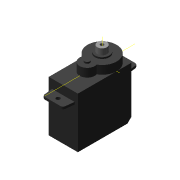
# Autodesk Inventor part: empty
Saved by Autodesk Inventor 2014 (Build 180170000, 170)
## iProperties
Created: 2015-04-13
Part Number: empty
Material: Generic
Document SubType Name: Modeling
Designer: Martin
Density: 1 g/cm^3
Appearance: Default
Author: Martin
Autodesk Inventor part; units mm, degrees
ref_plane "YZ Plane" through (0, 0, 0) normal (1, 0, 0) x (0, 1, 0)
ref_plane "XZ Plane" through (0, 0, 0) normal (0, 1, 0) x (-1, 0, 0)
sketch "Sketch1" plane through (0, 0, 0) normal (0, 0, 1) x (1, 0, 0)
  line L0 (-8.12, 0) -> (8.12, 0) projected
  line L1 (0, -19.7) -> (0, 10.05) projected
  circle A0 centre (0, 0) radius 5.8
  line L2 (-5.8, -15.45) -> (5.8, -15.45)
  line L3 (5.8, -15.45) -> (5.8, 5.8)
  line L4 (5.8, 5.8) -> (-5.8, 5.8)
  line L5 (-5.8, 5.8) -> (-5.8, -15.45)
  line L6 (-5.8, -15.45) -> (5.8, 5.8) construction
  line L7 (5.8, -15.45) -> (-5.8, 5.8) construction
  circle A1 centre (0, -5.95) radius 3
  point P0 (0, -4.825)
  point P1 (0, -8.95)
  dimension "d4" = 6
  dimension "d0" = 21.25
  dimension "d1" = 11.6
  dimension "d5" = 6.5
  constraints: 12 end point, 3 midpoint, 2 parallel, 2 point on line, 2 tangent, 1 centre point, 1 coincident, 1 horizontal, 1 perpendicular, 1 vertical alignment, 2 other
  measures "d0" distance between parallel lines of L2 L4
  measures "d1" distance of L2.start L2.end
  measures "d5" distance from line of L2 point (0, -8.95)
extrude "Extrusion1" add sketch "Sketch1" against normal blind 20.2
extrude "Extrusion2" add sketch "Sketch1" along normal blind 3.35 contours A0 L1 L0 | L0 L1 A1 A0 | L1 A0 L0 | L0 A0 A1 L1 | A1 L1 A0 | A0 L1 A1 | A1 A0 L1 | A0 A1 L1
sketch "Sketch2" plane through (0, 0, 3.35) normal (0, 0, 1) x (1, 0, 0)
  arc A0 (2.8604, -5.0456) -> (-2.8604, -5.0456) centre (0, 0) ccw projected
  arc A1 (-2.8604, -5.0456) -> (2.8604, -5.0456) centre (0, -5.95) ccw projected
  circle A2 centre (0, -5.95) radius 1
  circle A3 centre (0, 0) radius 2.85
  circle A4 centre (0, 0) radius 1.9
  circle A5 centre (0, 0) radius 1.875
  circle A6 centre (0, 0) radius 0.675
  dimension "d9" = 5.7
  dimension "d10" = 2
  dimension "d11" = 3.8
  dimension "d14" = 3.75
  dimension "d17" = 1.35
  constraints: 5 centre point, 5 coincident
  measures "d9" diameter of A3
  measures "d10" diameter of A2
  measures "d11" diameter of A4
  measures "d14" diameter of A5
  measures "d17" diameter of A6
extrude "Extrusion3" add sketch "Sketch2" along normal blind 0.6 contours A2 | A3
extrude "Extrusion4" add sketch "Sketch2" along normal blind 2.95 contours A5
ref_plane "Work Plane1" through (0, 0, -3.5) normal (0, 0, 1) x (1, 0, 0)
sketch "Sketch3" plane through (0, 0, -3.5) normal (0, 0, 1) x (1, 0, 0)
  line L0 (5.8, 5.8) -> (0, 5.8) projected
  line L1 (-5.8, 5.8) -> (5.8, 5.8) projected
  line L2 (0, 5.8) -> (-5.8, 5.8) projected
  line L3 (-5.8, -15.45) -> (5.8, -15.45) projected
  line L4 (5.8, -15.45) -> (-5.8, -15.45) projected
  line L5 (0, -19.7) -> (0, 10.05) projected
  line L6 (-5.8, 5.8) -> (-5.8, 0) projected
  line L7 (-5.8, -15.45) -> (-5.8, 5.8) projected
  line L8 (-5.8, 0) -> (-5.8, -15.45) projected
  line L9 (5.8, -15.45) -> (5.8, 0) projected
  line L10 (5.8, 5.8) -> (5.8, -15.45) projected
  line L11 (5.8, 0) -> (5.8, 5.8) projected
  line L12 (5.8, -4.825) -> (-5.8, -4.825)
  line L13 (-4.5, 5.8) -> (4.5, 5.8)
  line L14 (4.5, 5.8) -> (4, 10.05)
  line L15 (4, 10.05) -> (-4, 10.05)
  line L16 (-4, 10.05) -> (-4.5, 5.8)
  circle A0 centre (0, 7.875) radius 0.75
  line L17 (-4.5, -15.45) -> (4.5, -15.45)
  line L18 (4.5, -15.45) -> (4, -19.7)
  line L19 (4, -19.7) -> (-4, -19.7)
  line L20 (-4, -19.7) -> (-4.5, -15.45)
  circle A1 centre (0, -17.525) radius 0.75
  point P0 (0, 0)
  dimension "d19" = 1.5
  dimension "d20" = 9
  dimension "d21" = 8
  dimension "d22" = 4.25
  dimension "d23" = 25.4
  constraints: 18 end point, 7 point on line, 6 symmetric about line, 2 centre point, 2 parallel, 1 equal radius, 1 midpoint, 1 perpendicular, 1 other
  measures "d19" diameter of A0
  measures "d20" distance of L13.end L13.start
  measures "d21" distance of L14.end L15.end
  measures "d22" distance between parallel lines of L2 L15
  measures "d23" distance of A0.centre A1.centre
extrude "Extrusion5" add sketch "Sketch3" against normal blind 0.9 contours L0 L5 A0 L15 L14 | L1 L16 L15 L5 A0 | L5 A1 L19 L20 L3 | L3 L18 L19 L5 A1
fillet "Fillet1" radius 1 4 edges at (4, -19.7, -3.95) (-4, -19.7, -3.95) (4, 10.05, -3.95) (-4, 10.05, -3.95)
chamfer "Chamfer1" distance 1.5 angle 45 1 edges at (0, 5.8, -20.2)
sketch "Sketch4" plane through (0, 0, -4.4) normal (0, 0, -1) x (-1, 0, 0)
  arc A0 (4.1039, 9.1668) -> (3.1108, 10.05) centre (3.1108, 9.05) ccw projected
  line L0 (3.1108, 10.05) -> (-3.1108, 10.05) projected
  arc A1 (-3.1108, 10.05) -> (-4.1039, 9.1668) centre (-3.1108, 9.05) ccw projected
  line L1 (-4.1039, 9.1668) -> (-4.5, 5.8) projected
  line L2 (4.5, 5.8) -> (-4.5, 5.8) projected
  line L3 (4.5, 5.8) -> (4.1039, 9.1668) projected
  circle A2 centre (0, 7.875) radius 0.75 projected
  point P0 (0, 0)
extrude "BREAK_DA_TAB" [suppressed]
body "Solid1"
